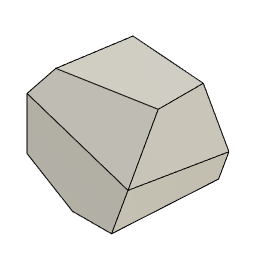
Suètone-stone (Autodesk Fusion 360 design; units mm, degrees)
Autodesk Fusion 360 part; units mm, degrees
ref_plane "Plan de construction7" through (0, 0, 3) normal (0, 0, 1) x (1, 0, 0)
sketch "Esquisse1" plane through (0, 0, 3) normal (0, 0, 1) x (1, 0, 0)
  line L0 (70, 70) -> (-70, 70)
  line L1 (-70, 70) -> (-70, -70)
  line L2 (-70, -70) -> (70, -70)
  line L3 (70, -70) -> (70, 70)
  line L4 (70, 70) -> (-70, -70) construction
  line L5 (-70, 70) -> (70, -70) construction
  line L6 (-70, -33.3126) -> (-7.049, -70)
  line L7 (-20, 70) -> (-70, 35)
  dimension "d1" = 140
  dimension "d2" = 140
  constraint horizontal L0
  constraint perpendicular L0 L1
  constraint parallel L0 L2
  constraint parallel L1 L3
  constraint coincident L4 origin
  constraint coincident L5 origin
  constraint coincident L1 L6.start
  constraint coincident L0 L7.start
  constraint coincident L1 L7.end
  constraint coincident L2 L6.end
  measures "d1" distance of L1.end L2.end
  measures "d2" distance of L0.end L1.end
extrude "Extrusion1" add sketch "Esquisse1" along normal blind 140 makes body 1
sketch "Esquisse3" plane through (0, 70, 0) normal (0, 1, 0) x (-1, 0, 0)
  line L0 (-70, 3) -> (70, 3)
  line L1 (70, 3) -> (70, 143)
  line L2 (70, 143) -> (-70, 143)
  line L3 (-70, 143) -> (-70, 3)
  line L4 (-70, 43) -> (70, 73)
  constraint coincident L3 L4.start
  constraint coincident L1 L4.end
  constraint midpoint L1 L4.end
ref_plane "Plan de construction1" through (0, 70, 58) normal (0.071663, 0.939693, 0.334428) x (-0.977802, 0, 0.209529)
split "Scinder1" by plane through (0, 70, 58) normal (0.071663, 0.939693, 0.334428) bodies 1 makes body 2 at (40, 70, 82.7619)
delete_body "RemoveBody1" bodies 2
sketch "Esquisse4" plane through (-70, 0, 0) normal (-1, 0, 0) x (0, -1, 0)
  line L0 (-45.0876, 143) -> (-70, 73)
  line L1 (-70, 73) -> (-70, 3)
  line L2 (-70, 3) -> (70, 3)
  line L3 (70, 3) -> (70, 143)
  line L4 (70, 143) -> (-45.0876, 143)
  line L5 (-70, 73) -> (70, 113)
  constraint coincident L0.end L1.start
  constraint coincident L3 L5.end
ref_plane "Plan de construction2" through (-70, 0, 93) normal (0.866025, -0.137361, -0.480762) x (0, -0.961524, 0.274721)
split "Scinder2" by plane through (-70, 0, 93) normal (0.866025, -0.137361, -0.480762) bodies 1 makes body 3 at (14.317, 23.3333, 3)
delete_body "RemoveBody2" bodies 1
sketch "Esquisse5" plane through (0, -70, 0) normal (0, -1, 0) x (1, 0, 0)
  line L0 (-53.3459, 143) -> (-70, 113)
  line L1 (-70, 113) -> (-70, 3)
  line L2 (-70, 3) -> (70, 3)
  line L3 (70, 3) -> (70, 143)
  line L4 (70, 143) -> (-53.3459, 143)
  line L5 (-70, 113) -> (70, 66.5695)
  constraint coincident L0.end L1.start
  constraint coincident L3 L5.end
ref_plane "Plan de construction3" through (0, -70, 89.7848) normal (-0.157393, 0.866025, -0.474581) x (0.949163, 0, -0.314786)
split "Scinder3" by plane through (0, -70, 89.7848) normal (-0.157393, 0.866025, -0.474581) bodies 3 makes body 4 at (14.317, 23.3333, 3)
delete_body "RemoveBody3" bodies 3
sketch "Esquisse6" plane through (70, 0, 0) normal (1, 0, 0) x (0, 1, 0)
  line L0 (-28.1162, 143) -> (-70, 66.5695)
  line L1 (-70, 66.5695) -> (-70, 3)
  line L2 (-70, 3) -> (70, 3)
  line L3 (70, 3) -> (70, 43)
  line L4 (70, 43) -> (34.4109, 143)
  line L5 (34.4109, 143) -> (-28.1162, 143)
  line L6 (70, 43) -> (-70, 66.5695)
  constraint coincident L3.end L4.start
  constraint coincident L0.end L1.start
ref_plane "Plan de construction4" through (70, 0, 54.7848) normal (0.939693, -0.056781, -0.337274) x (0, -0.986123, 0.166018)
split "Scinder4" by plane through (70, 0, 54.7848) normal (0.939693, -0.056781, -0.337274) bodies 4 makes body 5 at (70, -23.3333, 37.5232)
delete_body "RemoveBody4" bodies 5
ref_plane "Plan de construction5" through (-38.5245, -51.6563, 3) normal (0.38572, 0.661849, 0.642788) x (0.863982, -0.503522, 0)
split "Scinder5" by plane through (-38.5245, -51.6563, 3) normal (0.38572, 0.661849, 0.642788) bodies 4 makes body 6 at (9.5314, 23.3333, 3)
delete_body "RemoveBody5" bodies 4
ref_plane "Plan de construction6" through (-45, 52.5, 3) normal (0.405499, -0.579284, 0.707107) x (-0.819232, -0.573462, 0)
split "Scinder6" by plane through (-45, 52.5, 3) normal (0.405499, -0.579284, 0.707107) bodies 6 makes body 7 at (9.5314, 23.3333, 3)
delete_body "RemoveBody6" bodies 6
sketch "Esquisse7" plane through (0, 0, 3) normal (0, 0, 1) x (1, 0, 0)
  line L0 (-39.2516, 30.9727) -> (-45.0409, 35.541)
  line L1 (0, 0) -> (-50.7718, -26.722)
  line L2 (0, 0) -> (21.3084, -53.271)
  line L3 (0, 0) -> (54.0545, -19.2341)
  line L4 (19.1893, 46.1711) -> (22.0195, 52.981)
  line L5 (0, 0) -> (55.998, 12.4927)
  line L6 (0, 0) -> (-39.2516, 30.9727)
  arc A0 (-45.0409, 35.541) -> (-50.7718, -26.722) centre (0, 0) ccw construction
  line L7 (0, 0) -> (19.1893, 46.1711)
  arc A1 (21.3084, -53.271) -> (54.0545, -19.2341) centre (0, 0) ccw construction
  arc A2 (22.0195, 52.981) -> (-45.0409, 35.541) centre (0, 0) ccw
  arc A3 (55.998, 12.4927) -> (22.0195, 52.981) centre (0, 0) ccw construction
  arc A4 (54.0545, -19.2341) -> (55.998, 12.4927) centre (0, 0) ccw
  arc A5 (47.1067, -16.7619) -> (48.8003, 10.887) centre (0, 0) ccw
  arc A6 (48.8003, 10.887) -> (19.1893, 46.1711) centre (0, 0) ccw construction
  arc A7 (18.5695, -46.4238) -> (47.1067, -16.7619) centre (0, 0) ccw construction
  arc A8 (-39.2516, 30.9727) -> (-44.2459, -23.2873) centre (0, 0) ccw construction
  arc A9 (19.1893, 46.1711) -> (-39.2516, 30.9727) centre (0, 0) ccw
  arc A10 (-50.7718, -26.722) -> (21.3084, -53.271) centre (0, 0) ccw
  arc A11 (-44.2459, -23.2873) -> (18.5695, -46.4238) centre (0, 0) ccw
  constraint coincident L1.start L2.start
  constraint coincident L4.end A1
  constraint concentric A0 A1
  constraint concentric A1 A2
  constraint concentric A1 A3
  constraint concentric A1 A4
  constraint coincident L3 A5.start
  constraint coincident L5 A5.end
  constraint concentric A5 A6
  constraint coincident L1 A8.end
  constraint concentric A6 A7
  constraint concentric A6 A8
  constraint concentric A6 A9
  constraint concentric A1 A10
  constraint coincident L2 A7.start
  constraint concentric A7 A11
extrude "Extrusion2" [suppressed]
hole "Perçage1" at (-6.9679, 0.0504, 3) direction (0, 0, 1) diameter 100 depth 110 tip angle 180 bodies 7
sketch "Esquisse14" plane through (0, 0, 3) normal (0, 0, -1) x (1, 0, 0)
  circle A0 centre (-6.9679, -0.0504) radius 50
  line L0 (-70, -35) -> (-20, -70)
  line L1 (-20, -70) -> (55.6432, -70)
  line L2 (55.6432, -70) -> (47.1837, 70)
  line L3 (47.1837, 70) -> (-7.049, 70)
  line L4 (-7.049, 70) -> (-70, 33.3126)
  line L5 (-70, 33.3126) -> (-70, -35)
  line L6 (39.962, -64) -> (-0.038, -64)
  line L7 (-0.038, -64) -> (-0.038, -61)
  line L8 (-0.038, -61) -> (39.962, -61)
  line L9 (39.962, -61) -> (39.962, -64)
  line L10 (-61, -25) -> (-64, -25)
  line L11 (-64, -25) -> (-64, 15)
  line L12 (-64, 15) -> (-61, 15)
  line L13 (-61, 15) -> (-61, -25)
  line L14 (42, 65) -> (2, 65)
  line L15 (2, 65) -> (2, 62)
  line L16 (2, 62) -> (42, 62)
  line L17 (42, 62) -> (42, 65)
  dimension "d61" = 40
  dimension "d62" = 3
  dimension "d64" = 3
  dimension "d65" = 40
  dimension "d67" = 40
  dimension "d68" = 3
  constraint horizontal L6
  constraint vertical L7
  constraint horizontal L8
  constraint vertical L9
  constraint horizontal L10
  constraint vertical L11
  constraint horizontal L12
  constraint vertical L13
  constraint horizontal L14
  constraint vertical L15
  constraint horizontal L16
  constraint vertical L17
  measures "d61" distance of L6.start L6.end
  measures "d62" distance of L6.start L8.end
  measures "d64" distance of L10.start L10.end
  measures "d65" distance of L10.start L12.end
  measures "d67" distance of L14.start L14.end
  measures "d68" distance of L14.start L16.end
extrude "Extrusion9" add sketch "Esquisse14" along normal blind 3 separate body contours L6 L7 L8 L9 | L10 L11 L12 L13 | L14 L15 L16 L17 makes body 8 at (-64, 11.6667, 2) makes body 9 at (15.3333, -62, 2) makes body 10 at (26.6287, 64, 2)
ref_plane "Plan de construction8" through (-45, 52.5, 3) normal (0.573462, -0.819232, 0) x (0.819232, 0.573462, 0)
sketch "Esquisse18" plane through (0, 0, 3) normal (0, 0, -1) x (1, 0, 0)
  circle A0 centre (-6.9679, -0.0504) radius 50
  line L0 (-70, -35) -> (-20, -70)
  line L1 (-20, -70) -> (55.6432, -70)
  line L2 (55.6432, -70) -> (47.1837, 70)
  line L3 (47.1837, 70) -> (-7.049, 70)
  line L4 (-7.049, 70) -> (-70, 33.3126)
  line L5 (-70, 33.3126) -> (-70, -35)
  line L6 (-6.9679, -0.0504) -> (-6.9679, 49.9496) construction
  line L7 (-6.9679, -0.0504) -> (-6.9679, -50.0504) construction
  line L8 (-6.9679, -0.0504) -> (-56.9679, -0.0504) construction
  line L9 (-6.9679, -0.0504) -> (43.0321, -0.0504) construction
  line L10 (0.5321, 59.9496) -> (-14.4679, 59.9496)
  line L11 (-14.4679, 59.9496) -> (-14.4679, -60.0504)
  line L12 (-14.4679, -60.0504) -> (0.5321, -60.0504)
  line L13 (0.5321, -60.0504) -> (0.5321, 59.9496)
  line L14 (0.5321, 59.9496) -> (-14.4679, -60.0504) construction
  line L15 (-14.4679, 59.9496) -> (0.5321, -60.0504) construction
  circle A1 centre (-7, -55) radius 1.75
  circle A2 centre (-6.9679, 55.0242) radius 1.75
  point P0 (-6.9679, -0.0504)
  dimension "d82" = 15
  dimension "d83" = 120
  dimension "d86" = 3.5
  dimension "d87" = 3.5
  constraint coincident P0 A0.centre
  constraint coincident A0 L6.end
  constraint perpendicular L3 L6
  constraint coincident A0 L7.end
  constraint perpendicular L3 L7
  constraint coincident A0 L8.end
  constraint perpendicular L6 L8
  constraint coincident A0 L9.end
  constraint perpendicular L6 L9
  constraint horizontal L10
  constraint perpendicular L10 L11
  constraint parallel L10 L12
  constraint parallel L11 L13
  constraint coincident L14 P0
  constraint coincident L15 P0
  measures "d82" distance of L11.end L12.end
  measures "d83" distance of L10.end L11.end
  measures "d86" diameter of A1
  measures "d87" diameter of A2
sketch "Esquisse20" plane through (-39.4631, 56.3758, 0) normal (0.573462, -0.819232, 0) x (0.819232, 0.573462, 0)
sketch "Esquisse21" plane through (-39.4631, 56.3758, 0) normal (0.573462, -0.819232, 0) x (0.819232, 0.573462, 0)
  circle A0 centre (-11.9845, 13.6214) radius 6
  dimension "d79" = 12
  measures "d79" diameter of A0
extrude "Extrusion10" cut sketch "Esquisse21" along normal mid plane 44 bodies 7
extrude "Extrusion11" cut sketch "Esquisse18" against normal blind 5 contours A0 L10 L11 L13 | A0 L11 L12 L13 | A1 | A2 bodies 7
extrude "Extrusion12" cut sketch "Esquisse18" against normal blind 20 contours A1 | A2 bodies 7
sketch "Esquisse23" plane through (0, 0, 3) normal (0, 0, -1) x (1, 0, 0)
shell "Coque1" [suppressed]
sketch "Esquisse9" plane through (-65, 0, 0) normal (1, 0, 0) x (0, 1, 0)
  line L0 (19.9112, 3) -> (65, 39.0711)
  line L1 (65, 39.0711) -> (65, 70.5584)
  line L2 (65, 70.5584) -> (63.6689, 72.9162)
  line L3 (63.6689, 72.9162) -> (-65, 109.6788)
  line L4 (-65, 109.6788) -> (-65, 50.9548)
  line L5 (-65, 50.9548) -> (-15.5503, 3)
  line L6 (-15.5503, 3) -> (19.9112, 3)
  line L7 (-15.5503, 3) -> (19.9112, 3)
  line L8 (19.9112, 3) -> (19.9112, 8)
  line L9 (19.9112, 8) -> (-15.5503, 8)
  line L10 (-15.5503, 8) -> (-15.5503, 3)
  dimension "d21" = 5
  constraint horizontal L7
  constraint vertical L8
  constraint horizontal L9
  constraint vertical L10
  constraint coincident L6 L5.end
  constraint coincident L0.start L6.end
  measures "d21" distance of L8.end L0.start
extrude "Extrusion5" [suppressed]
fillet "Congé2" [suppressed]
fillet "Congé3" [suppressed]
sketch "Esquisse11" plane through (0, 0, 0) normal (0, 1, 0) x (1, 0, 0)
  line L0 (-4.8816, -3, 65) -> (-4.8816, -8, 65)
  line L1 (-4.8816, -8, 65) -> (48.6854, -8, 65)
  line L2 (50.0202, -3, 65) -> (-4.8816, -3, 65)
  line L3 (48.6854, -8, 65) -> (48.6854, -3, 65)
  point P0 (-4.8816, -3)
  dimension "d29" = 5
extrude "Extrusion6" [suppressed]
fillet "Congé4" [suppressed]
fillet "Congé5" [suppressed]
sketch "Esquisse12" plane through (0, -65, 0) normal (0, 1, 0) x (-1, 0, 0)
  line L0 (-4.2295, 3) -> (65, 50.9548)
  line L1 (65, 50.9548) -> (65, 109.6788)
  line L2 (65, 109.6788) -> (64.8399, 109.8772)
  line L3 (64.8399, 109.8772) -> (-65, 66.8163)
  line L4 (-65, 66.8163) -> (-65, 66.6218)
  line L5 (-65, 66.6218) -> (-42.1649, 3)
  line L6 (-42.1649, 3) -> (-4.2295, 3)
  line L7 (-4.2295, 3) -> (-4.2295, 8)
  line L8 (-4.2295, 8) -> (-40.2295, 8)
  line L9 (-40.2295, 8) -> (-40.2295, 3)
  dimension "d36" = 5
  dimension "d37" = 36
  constraint coincident L0.start L6.end
  constraint perpendicular L6 L7
  constraint horizontal L8
  constraint coincident L6 L9.end
  constraint perpendicular L6 L9
  measures "d36" distance of L0.start L7.end
  measures "d37" distance of L7.end L8.end
extrude "Extrusion7" [suppressed]
fillet "Congé6" [suppressed]
fillet "Congé7" [suppressed]
sketch "Esquisse13" plane through (0, 0, 3) normal (0, 0, -1) x (1, 0, 0)
  arc A0 (37.2295, 55) -> (40.2295, 58) centre (37.2295, 58) ccw
  line L0 (40.2295, 58) -> (40.2295, 65)
  line L1 (40.2295, 65) -> (42.1649, 65)
  line L2 (42.1649, 65) -> (50.0202, -65)
  line L3 (50.0202, -65) -> (48.6854, -65)
  line L4 (48.6854, -65) -> (48.6854, -58)
  arc A1 (48.6854, -58) -> (45.6854, -55) centre (45.6854, -58) ccw
  line L5 (45.6854, -55) -> (-1.8816, -55)
  arc A2 (-1.8816, -55) -> (-4.8816, -58) centre (-1.8816, -58) ccw
  line L6 (-4.8816, -58) -> (-4.8816, -65)
  line L7 (-4.8816, -65) -> (-65, -19.9112)
  line L8 (-65, -19.9112) -> (-58, -19.9112)
  arc A3 (-58, -19.9112) -> (-55, -16.9112) centre (-58, -16.9112) ccw
  line L9 (-55, -16.9112) -> (-55, 12.5503)
  arc A4 (-55, 12.5503) -> (-58, 15.5503) centre (-58, 12.5503) ccw
  line L10 (-58, 15.5503) -> (-65, 15.5503)
  line L11 (-65, 15.5503) -> (4.2295, 65)
  line L12 (4.2295, 65) -> (4.2295, 58)
  arc A5 (4.2295, 58) -> (7.2295, 55) centre (7.2295, 58) ccw
  line L13 (7.2295, 55) -> (37.2295, 55)
  line L14 (-70, -25) -> (-10, -70)
  line L15 (-10, -70) -> (55.6432, -70)
  line L16 (55.6432, -70) -> (47.1837, 70)
  line L17 (47.1837, 70) -> (0, 70)
  line L18 (0, 70) -> (-70, 20)
  line L19 (-70, 20) -> (-70, -25)
  line L20 (44.5121, -63) -> (-0.4879, -63)
  line L21 (-0.4879, -63) -> (-0.4879, -58)
  line L22 (-0.4879, -58) -> (44.5121, -58)
  line L23 (44.5121, -58) -> (44.5121, -63)
  line L24 (-58.4932, -17.4547) -> (-63.4932, -17.4547)
  line L25 (-63.4932, -17.4547) -> (-63.4932, 12.5453)
  line L26 (-63.4932, 12.5453) -> (-58.4932, 12.5453)
  line L27 (-58.4932, 12.5453) -> (-58.4932, -17.4547)
  line L28 (37, 58) -> (7, 58)
  line L29 (7, 58) -> (7, 63)
  line L30 (7, 63) -> (37, 63)
  line L31 (37, 63) -> (37, 58)
  dimension "d44" = 45
  dimension "d45" = 5
  dimension "d46" = 5
  dimension "d47" = 30
  dimension "d48" = 30
  dimension "d49" = 5
  constraint horizontal L20
  constraint vertical L21
  constraint horizontal L22
  constraint vertical L23
  constraint horizontal L24
  constraint vertical L25
  constraint horizontal L26
  constraint vertical L27
  constraint horizontal L28
  constraint vertical L29
  constraint horizontal L30
  constraint vertical L31
  measures "d44" distance of L20.start L20.end
  measures "d45" distance of L20.start L22.end
  measures "d46" distance of L24.start L24.end
  measures "d47" distance of L24.start L26.end
  measures "d48" distance of L28.start L28.end
  measures "d49" distance of L28.start L30.end
extrude "Extrusion8" [suppressed]
fillet "Congé8" [suppressed]
fillet "Congé9" [suppressed]
fillet "Congé10" [suppressed]
